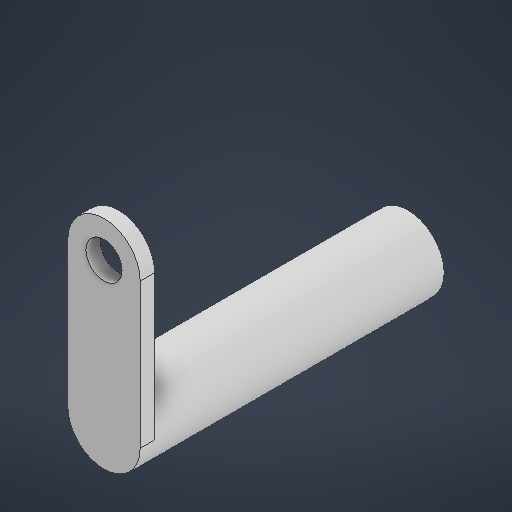
# Autodesk Inventor part: main rack connection
Saved by Autodesk Inventor 2026.1 (Build 301233000, 233)
## iProperties
Created: 2026-06-10
Part Number: main rack connection
Material: Generic
Document SubType Name: Modeling
Designer: share
Density: 1 g/cm^3
Appearance: Default
Author: share
Autodesk Inventor part; units mm, degrees
ref_plane "YZ Plane" through (0, 0, 0) normal (1, 0, 0) x (0, 1, 0)
ref_plane "XZ Plane" through (0, 0, 0) normal (0, 1, 0) x (-1, 0, 0)
ref_plane "XY Plane" through (0, 0, 0) normal (0, 0, 1) x (1, 0, 0)
sketch "Sketch1" plane through (0, 0, 0) normal (0, 0, 1) x (1, 0, 0)
  circle A0 centre (0, 0) radius 6.35
  dimension "d0" = 12.7
  constraints: 1 centre point, 1 coincident
  measures "d0" diameter of A0
extrude "Extrusion1" add sketch "Sketch1" along normal blind 50.8
sketch "Sketch2" plane through (0, 0, 50.8) normal (0, 0, 1) x (1, 0, 0)
  circle A0 centre (0, 0) radius 6.35 projected
  line L0 (0, 0) -> (0, 25.4)
  circle A1 centre (0, 25.4) radius 6.35
  line L1 (-6.35, 25.4) -> (-6.35, 0)
  line L2 (6.35, 25.4) -> (6.35, 0)
  circle A2 centre (0, 25.4) radius 3.175
  dimension "d3" = 25.4
  dimension "d6" = 6.35
  constraints: 6 end point, 4 point on circle, 3 tangent, 2 centre point, 2 coincident, 1 equal radius, 1 parallel, 1 vertical
  measures "d3" distance of L0.start L0.end
  measures "d6" diameter of A2
extrude "Extrusion2" add sketch "Sketch2" along normal blind 2.54
body "Solid1"
